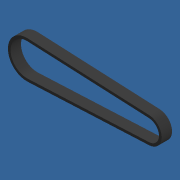
# Autodesk Inventor part: Bed_Unit_Belt
Saved by Autodesk Inventor 2020 (Build 240168000, 168)
## iProperties
Created: 2020-10-05
Part Number: Bed_Unit_Belt
Material: ゴム
Document SubType Name: Modeling
Designer: kenta iguchi
Density: 0.93 g/cm^3
Appearance: ゴム - 黒
Author: kenta iguchi
Autodesk Inventor part; units mm, degrees
ref_plane "YZ Plane" through (0, 0, 0) normal (1, 0, 0) x (0, 1, 0)
ref_plane "XZ Plane" through (0, 0, 0) normal (0, 1, 0) x (-1, 0, 0)
ref_plane "XY Plane" through (0, 0, 0) normal (0, 0, 1) x (1, 0, 0)
sketch "スケッチ1" plane through (0, 0, 0) normal (0, 0, 1) x (1, 0, 0)
  arc A0 (0.4385, 9.2897) -> (0.4384, -9.2897) centre (0, 0) ccw
  arc A1 (0.5091, 10.788) -> (0.5091, -10.788) centre (0, 0) ccw
  arc A2 (70.3536, -7.4917) -> (70.3536, 7.4917) centre (70, 0) ccw
  line L0 (0.5091, 10.788) -> (70.3536, 7.4917)
  line L1 (70.3536, -7.4917) -> (0.5091, -10.788)
  line L2 (70.1922, 5.9969) -> (0.4385, 9.2897)
  circle A3 centre (70, 0) radius 6
  line L3 (0.4384, -9.2897) -> (70.2829, -5.9933)
  point P0 (1.0111, -13.9634)
  point P1 (90.5417, -7.4804)
  point P2 (90.5417, 7.4804)
  point P3 (1.0111, 13.9634)
  point P4 (0.9028, 12.4674)
  dimension "d0" = 18.6
  dimension "d2" = 70
  dimension "d3" = 1.5
  dimension "d7" = 12
  dimension "d8" = 1.5
  constraints: 8 end point, 8 point on circle, 7 tangent, 4 centre point, 2 coincident, 1 horizontal alignment
  measures "d0" diameter of A0
  measures "d2" distance of point (0, 0) A2.centre
  measures "d3" radial gap between concentric circles of A0 A1
  measures "d7" diameter of A3
  measures "d8" radial gap between concentric circles of A2 A3
extrude "押し出し1" add sketch "スケッチ1" along normal blind 6
